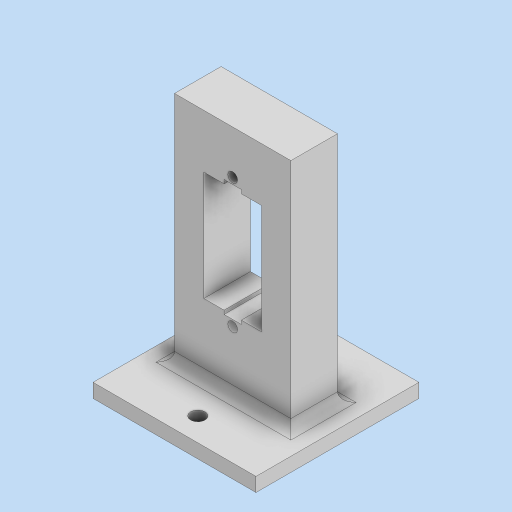
# Autodesk Inventor part: base de motor
Saved by Autodesk Inventor 2024 (Build 280153000, 153)
## iProperties
Created: 2024-09-04
Part Number: base de motor
Material: Generic
Document SubType Name: Modeling
Designer: MxMon
Density: 1 g/cm^3
Appearance: Default
Author: MxMon
Autodesk Inventor part; units mm, degrees
ref_plane "YZ Plane" through (0, 0, 0) normal (1, 0, 0) x (0, 1, 0)
ref_plane "XZ Plane" through (0, 0, 0) normal (0, 1, 0) x (-1, 0, 0)
ref_plane "XY Plane" through (0, 0, 0) normal (0, 0, 1) x (1, 0, 0)
sketch "Sketch1" plane through (0, 0, 0) normal (0, 1, 0) x (-1, 0, 0)
  line L0 (-17.5, -17.5) -> (17.5, -17.5)
  line L1 (17.5, -17.5) -> (17.5, 17.5)
  line L2 (17.5, 17.5) -> (-17.5, 17.5)
  line L3 (-17.5, 17.5) -> (-17.5, -17.5)
  line L4 (-17.5, -17.5) -> (17.5, 17.5) construction
  line L5 (17.5, -17.5) -> (-17.5, 17.5) construction
  point P0 (0, 0)
  dimension "d0" = 35
  dimension "d1" = 35
  constraints: 12 end point, 2 midpoint, 2 parallel, 1 horizontal, 1 perpendicular
  measures "d0" distance of L2.end L1.end
  measures "d1" distance of L1.end L0.end
extrude "Extrusion1" add sketch "Sketch1" along normal blind 3
sketch "Sketch2" plane through (0, 3, 0) normal (0, 1, 0) x (1, 0, 0)
  line L0 (-12.5, 5) -> (12.5, 5)
  line L1 (12.5, 5) -> (12.5, -5)
  line L2 (12.5, -5) -> (-12.5, -5)
  line L3 (-12.5, -5) -> (-12.5, 5)
  line L4 (-12.5, 5) -> (12.5, -5) construction
  line L5 (12.5, 5) -> (-12.5, -5) construction
  point P0 (0, 0)
  dimension "d4" = 25
  dimension "d5" = 10
  constraints: 12 end point, 2 midpoint, 2 parallel, 1 horizontal, 1 perpendicular
  measures "d4" distance of L0.start L0.end
  measures "d5" distance of L2.end L0.start
extrude "Extrusion2" add sketch "Sketch2" along normal blind 50
sketch "Sketch3" plane through (-12.5, 3, 5) normal (0, 0, 1) x (1, 0, 0)
  line L0 (6.3, 38.5) -> (18.7, 38.5)
  line L1 (18.7, 38.5) -> (18.7, 15)
  line L2 (18.7, 15) -> (6.3, 15)
  line L3 (6.3, 15) -> (6.3, 38.5)
  line L4 (6.3, 38.5) -> (18.7, 15) construction
  line L5 (18.7, 38.5) -> (6.3, 15) construction
  line L6 (-5, 0) -> (30, 0) projected
  line L7 (0, 50) -> (25, 50) projected
  point P0 (12.5, -3)
  point P1 (12.5, 26.75)
  point P2 (12.5, 38.5)
  point P3 (12.5, 50)
  dimension "d8" = 12.4
  dimension "d9" = 23.5
  dimension "d10" = 15
  constraints: 12 end point, 4 midpoint, 2 parallel, 1 horizontal, 1 perpendicular, 1 vertical alignment
  measures "d8" distance of L1.end L2.end
  measures "d9" distance of L0.end L1.end
  measures "d10" distance between parallel lines of L2 L6
fillet "Fillet1" radius 2 4 edges at (-12.5, 3, 0) (12.5, 3, 0) (0, 3, 5) (0, 3, -5)
extrude "Extrusion4" cut sketch "Sketch3" against normal through all
sketch "Sketch5" plane through (-12.5, 53, 5) normal (0, 0, 1) x (1, 0, 0)
  circle A0 centre (12.5, -9.35) radius 1.05
  line L0 (6.3, -11.5) -> (18.7, -11.5) projected
  line L1 (18.7, -11.5) -> (18.7, -35) construction
  line L2 (18.7, -23.25) -> (6.3, -23.25) construction
  circle A1 centre (12.5, -37.15) radius 1.05
  point P0 (12.5, -53)
  point P1 (12.5, -11.5)
  point P2 (12.5, -11.5)
  dimension "d18" = 2.1
  dimension "d19" = 2.15
  constraints: 3 midpoint, 2 centre point, 2 end point, 1 horizontal, 1 symmetric about line, 1 vertical alignment, 1 other
  measures "d18" diameter of A0
  measures "d19" distance of point (12.5, -11.5) A0.centre
extrude "Extrusion5" cut sketch "Sketch5" against normal blind 10
sketch "Sketch6" plane through (-6.2, 41.5, 5) normal (0, -1, 0) x (1, 0, 0)
  line L0 (12.4, 0) -> (12.4, -10) projected
  line L1 (0, 0) -> (0, -10) projected
  line L2 (0, 0) -> (12.4, 0) projected
  line L3 (12.4, -10) -> (0, -10) projected
  line L4 (8.05, -10) -> (4.35, -10)
  line L5 (4.35, -10) -> (4.35, 0)
  line L6 (4.35, 0) -> (8.05, 0)
  line L7 (8.05, 0) -> (8.05, -10)
  line L8 (8.05, -10) -> (4.35, 0) construction
  line L9 (4.35, -10) -> (8.05, 0) construction
  point P0 (6.2, -5)
  point P1 (6.2, -5)
  point P2 (6.2, -10)
  point P3 (6.2, -10)
  point P4 (8.05, -5)
  point P5 (12.4, -5)
  point P6 (8.05, 0)
  point P7 (4.35, 0)
  point P8 (4.35, -10)
  dimension "d22" = 3.7
  dimension "d23" = 10
  constraints: 12 end point, 6 midpoint, 2 parallel, 1 coincident, 1 horizontal, 1 horizontal alignment, 1 perpendicular
  measures "d22" distance of L5.end L6.end
  measures "d23" distance of L4.end L5.end
extrude "Extrusion6" cut sketch "Sketch6" against normal blind 0.8 contours L7 L3 L5 L2
sketch "Sketch8" plane through (0, 0, 0) normal (0, -1, 0) x (1, 0, 0)
  line L0 (-17.5, 17.5) -> (17.5, 17.5) projected
  point P0 (0, 0)
  point P1 (0, 12.5)
  dimension "d41" = 5
  constraints: 1 vertical alignment
  measures "d41" distance from line of L0 point (0, 12.5)
hole "Hole2" at (0, 0, 12.5) direction (0, 1, 0) diameter 3.1 end through all
mirror "Mirror3" about plane through (0, 0, 0) normal (0, 0, 1) of "Hole2"
sketch "Sketch9" plane through (-6.2, 18, 5) normal (0, 1, 0) x (1, 0, 0)
  line L0 (4.35, 10) -> (4.35, 0) projected
  line L1 (8.05, 0) -> (8.05, 10) projected
  line L2 (4.35, 0) -> (8.05, 0) projected
  line L3 (8.05, 10) -> (4.35, 10) projected
  point P0 (6.2, 5)
extrude "Extrusion7" cut sketch "Sketch9" against normal blind 0.8
body "Solid1"
